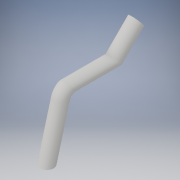
# Autodesk Inventor part: rocker (1.1)
Saved by Autodesk Inventor 2017 (Build 210142000, 142)
## iProperties
Created: 2017-10-27
Part Number: rocker (1.1)
Material: Generic
Document SubType Name: Modeling
Designer: 602199
Density: 1 g/cm^3
Appearance: Default
Author: 602199
Autodesk Inventor part; units mm, degrees
ref_plane "YZ Plane" through (0, 0, 0) normal (1, 0, 0) x (0, 1, 0)
ref_plane "XZ Plane" through (0, 0, 0) normal (0, 1, 0) x (-1, 0, 0)
ref_plane "XY Plane" through (0, 0, 0) normal (0, 0, 1) x (1, 0, 0)
sketch "Sketch1" plane through (0, 0, 0) normal (0, 1, 0) x (-1, 0, 0)
  circle A0 centre (0, 0) radius 19.05
  dimension "d0" = 38.1
  constraints: 1 centre point, 1 coincident
  measures "d0" diameter of A0
sketch "Sketch2" plane through (0, 0, 0) normal (1, 0, 0) x (0, 1, 0)
  line L0 (0, 0) -> (139.7, -38.1128)
  line L1 (0, 0) -> (144.8056, 0) construction
  dimension "d4" = 15.26
  constraints: 4 end point, 1 equal length, 1 horizontal
  measures "d4" angle of L0 L1
sweep "Sweep1" add profiles "Sketch1" path "Sketch2"
sketch "Sketch3" plane through (0, 139.7, -38.1128) normal (0, 1, 0) x (1, 0, 0)
  circle A0 centre (0, 0) radius 19.05
  point P0 (0, -38.1128)
  constraints: 1 centre point
sketch "Sketch4" plane through (0, 0, 0) normal (1, 0, 0) x (0, 1, 0)
  line L0 (139.7, -57.1628) -> (139.7, -19.0628) projected
  arc A0 (158.75, -57.1628) -> (139.7, -38.1128) centre (130.214, -66.6487) ccw
  line L1 (158.75, -184.1628) -> (260.35, -184.1628) construction
  point P0 (0, 0)
  constraints: 2 end point, 2 point on circle, 1 centre point, 1 horizontal, 1 midpoint
sweep "Sweep2" add profiles "Sketch3" path "Sketch4" path curves A0
sketch "Sketch5" plane through (0, 158.75, -57.1628) normal (0, 0.5986852, -0.8009844) x (-1, 0, 0)
  circle A0 centre (0, 0) radius 19.05
  point P0 (0, -92.9338)
  constraints: 1 centre point
sketch "Sketch6" plane through (0, 0, 0) normal (1, 0, 0) x (0, 1, 0)
  line L0 (158.75, -57.1628) -> (158.75, -184.1628)
  point P0 (0, 0)
  dimension "d16" = 127
  constraints: 2 end point, 1 vertical
  measures "d16" distance of L0.start L0.end
sweep "Sweep3" add profiles "Sketch5" path "Sketch6"
sketch "Sketch7" plane through (0, 158.75, -184.1628) normal (0, 0.5986852, -0.8009844) x (-1, 0, 0)
  circle A0 centre (0, 0) radius 19.05
  point P0 (0, -16.9007)
  constraints: 1 centre point
sketch "Sketch8" plane through (0, 0, 0) normal (1, 0, 0) x (0, 1, 0)
  line L0 (143.4912, -195.5677) -> (174.0088, -172.7578) projected
  line L1 (158.75, -184.1628) -> (220.955, -246.3677)
  line L2 (158.75, -184.1628) -> (246.7211, -184.1628) construction
  point P0 (0, 0)
  dimension "d20" = 45
  constraints: 4 end point, 1 equal length, 1 horizontal
  measures "d20" angle of L1 L2
sweep "Sweep4" add profiles "Sketch7" path "Sketch8" path curves L1
sketch "Sketch13" plane through (0, 0, 0) normal (1, 0, 0) x (0, 1, 0)
  line L0 (205.6962, -257.7727) -> (236.2137, -234.9628) projected
  point P0 (0, 0)
body "Solid1"
